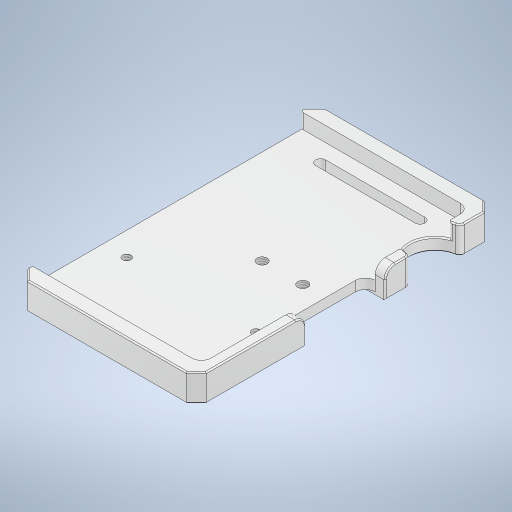
# Autodesk Inventor part: Wallet Recipe Test
Saved by Autodesk Inventor 2023.2 (Build 272271000, 271)
## iProperties
Created: 2024-03-26
Part Number: Wallet Recipe Test
Material: Aluminum 6061
Document SubType Name: Modeling
Designer: Nathan Cai
Density: 2.7 g/cm^3
Appearance: Aluminum - Flat
Author: Nathan Cai
Autodesk Inventor part; units mm, degrees
ref_plane "YZ Plane" through (0, 0, 0) normal (1, 0, 0) x (0, 1, 0)
ref_plane "XZ Plane" through (0, 0, 0) normal (0, 1, 0) x (-1, 0, 0)
ref_plane "XY Plane" through (0, 0, 0) normal (0, 0, 1) x (1, 0, 0)
sketch "Sketch1" plane through (0, 0, 0) normal (0, 1, 0) x (-1, 0, 0)
  line L0 (-28.575, 47.625) -> (28.575, 47.625)
  line L1 (28.575, 47.625) -> (28.575, -47.625)
  line L2 (28.575, -47.625) -> (-28.575, -47.625)
  line L3 (-28.575, -47.625) -> (-28.575, 47.625)
  line L4 (-28.575, 47.625) -> (28.575, -47.625) construction
  line L5 (28.575, 47.625) -> (-28.575, -47.625) construction
  point P0 (0, 0)
  dimension "d0" = 57.15
  dimension "d1" = 95.25
  constraints: 12 end point, 2 midpoint, 2 parallel, 1 horizontal, 1 perpendicular
  measures "d0" distance of L1.end L2.end
  measures "d1" distance of L0.end L1.end
extrude "Extrusion1" add sketch "Sketch1" along normal blind 8.7313
sketch "Sketch2" plane through (0, 8.7313, 0) normal (0, 1, 0) x (1, 0, 0)
  line L0 (-28.575, 47.625) -> (-28.575, -47.625) projected
  line L1 (-28.575, 0) -> (0, 0) construction
  line L2 (-28.575, -42.8625) -> (25.4, -42.8625)
  line L3 (25.4, -42.8625) -> (25.4, 42.8625)
  line L4 (25.4, 42.8625) -> (-28.575, 42.8625)
  line L5 (-28.575, 42.8625) -> (-28.575, -42.8625)
  dimension "d4" = 53.975
  dimension "d5" = 85.725
  constraints: 10 end point, 2 horizontal, 2 parallel, 1 midpoint, 1 perpendicular, 1 point on line, 1 other
  measures "d4" distance of L4.end L3.end
  measures "d5" distance of L3.end L2.end
extrude "Extrusion2" cut sketch "Sketch2" against normal blind 4.7625
fillet "Fillet1" radius 3.048 2 edges at (25.4, 6.35, 42.8625) (25.4, 6.35, -42.8625)
sketch "Sketch3" plane through (0, 0, 0) normal (0, -1, 0) x (1, 0, 0)
  line L0 (22.225, -12.7) -> (34.925, -12.7)
  line L1 (34.925, -12.7) -> (34.925, 12.7)
  line L2 (34.925, 12.7) -> (22.225, 12.7)
  line L3 (22.225, 12.7) -> (22.225, -12.7)
  line L4 (28.575, 47.625) -> (28.575, -47.625) projected
  line L5 (22.225, -12.7) -> (34.925, 12.7) construction
  line L6 (34.925, -12.7) -> (22.225, 12.7) construction
  point P0 (0, 0)
  point P1 (28.575, 0)
  dimension "d15" = 12.7
  dimension "d16" = 25.4
  constraints: 12 end point, 3 midpoint, 2 parallel, 1 horizontal, 1 perpendicular
  measures "d15" distance of L2.end L1.end
  measures "d16" distance between parallel lines of L0 L2
extrude "Extrusion3" cut sketch "Sketch3" against normal through all
sketch "Sketch4" plane through (0, 0, 0) normal (0, -1, 0) x (1, 0, 0)
  line L0 (28.575, -12.7) -> (-19.05, -12.7)
  line L1 (-19.05, -12.7) -> (-19.05, 12.7)
  line L2 (-19.05, 12.7) -> (28.575, 12.7)
  line L3 (28.575, 12.7) -> (28.575, -12.7)
  line L4 (28.575, -12.7) -> (-19.05, 12.7) construction
  line L5 (-19.05, -12.7) -> (28.575, 12.7) construction
  line L6 (0, 0) -> (22.225, 0) construction
  line L7 (22.225, 12.7) -> (22.225, -12.7) projected
  point P0 (4.7625, 0)
  point P1 (28.575, 12.7)
  point P2 (22.225, 9.525)
  point P3 (22.225, -9.525)
  dimension "d20" = 47.625
  dimension "d21" = 25.4
  constraints: 14 end point, 3 midpoint, 2 parallel, 2 point on line, 1 horizontal, 1 perpendicular
  measures "d20" distance of L1.end L2.end
  measures "d21" distance of L0.end L1.end
extrude "Extrusion4" cut sketch "Sketch4" against normal blind 0.7937
fillet "Fillet3" radius 3.175 6 edges at (22.225, 2.3813, -12.7) (26.9875, 8.7313, -12.7) (22.225, 2.3813, 12.7) (26.9875, 8.7313, 12.7) (-19.05, 0.3969, -12.7) (-19.05, 0.3969, 12.7)
sketch "Sketch5" plane through (0, 0.7937, 0) normal (0, -1, 0) x (1, 0, 0)
  line L0 (-19.05, -9.525) -> (-19.05, 9.525) projected
  line L1 (-19.05, 0) -> (22.225, 0) construction
  line L2 (22.225, 9.525) -> (22.225, -9.525) projected
  circle A0 centre (1.95, 0) radius 2
  circle A1 centre (14.95, 0) radius 2
  point P0 (0, 0)
  dimension "d25" = 4
  dimension "d26" = 21
  dimension "d29" = 13
  constraints: 2 centre point, 2 coincident, 2 end point, 2 midpoint, 1 horizontal, 1 point on line, 2 other
  measures "d25" diameter of A0
  measures "d26" distance from line of L0 A0.centre
  measures "d29" distance of A0.centre A1.centre
hole "Hole1" at (1.95, 0.7937, 0) at (14.95, 0.7937, 0) direction (0, 1, 0) diameter 3.242 end through all thread size "M4x0.7" class "6H" standard "ANSI Metric M Profile"
chamfer "Chamfer3" distance 3.175 angle 45 4 edges at (28.575, 4.3656, 47.625) (-28.575, 4.3656, 47.625) (28.575, 4.3656, -47.625) (-28.575, 4.3656, -47.625)
fillet "Fillet4" radius 0.7937 2 edges at (-28.575, 6.35, 42.8625) (-28.575, 6.35, -42.8625)
sketch "Sketch7" plane through (0, 0, 0) normal (0, -1, 0) x (1, 0, 0)
  line L0 (25.4, -47.625) -> (-25.4, -47.625) projected
  line L1 (0, -47.625) -> (0, 47.625) construction
  line L2 (-25.4, 47.625) -> (25.4, 47.625) projected
  line L3 (15.875, -36.5125) -> (-15.875, -36.5125) construction
  line L4 (15.875, -34.925) -> (-15.875, -34.925)
  line L5 (-15.875, -38.1) -> (15.875, -38.1)
  arc A0 (15.875, -38.1) -> (15.875, -34.925) centre (15.875, -36.5125) ccw
  arc A1 (-15.875, -34.925) -> (-15.875, -38.1) centre (-15.875, -36.5125) ccw
  line L6 (28.575, -12.7) -> (28.575, -44.45) projected
  circle A2 centre (28.575, -28.575) radius 7.9375
  point P0 (0, 0)
  point P1 (0, -36.5125)
  point P2 (28.575, -36.5125)
  point P3 (28.575, -20.6375)
  dimension "d50" = 3.175
  dimension "d51" = 31.75
  dimension "d52" = 9.525
  dimension "d55" = 15.875
  constraints: 10 end point, 4 midpoint, 4 point on circle, 4 tangent, 3 centre point, 1 parallel, 1 perpendicular, 1 point on line
  measures "d50" diameter of A1
  measures "d51" distance of L3.start L3.end
  measures "d52" distance between parallel lines of L0 L5
  measures "d55" diameter of A2
extrude "Extrusion6" cut sketch "Sketch7" against normal blind 25.4 contours A0 L5 A1 L4 | L6 A2 picked at (24.9577, -30.7816)
sketch "Sketch8" plane through (0, 0, 0) normal (0, -1, 0) x (1, 0, 0)
  line L0 (0, 0) -> (0, 47.625) construction
  line L1 (-25.4, 47.625) -> (25.4, 47.625) construction
  line L2 (-23.8125, 17.4625) -> (23.8125, 17.4625)
  line L3 (23.8125, 17.4625) -> (23.8125, 42.8625)
  line L4 (23.8125, 42.8625) -> (-23.8125, 42.8625)
  line L5 (-23.8125, 42.8625) -> (-23.8125, 17.4625)
  line L6 (-23.8125, 17.4625) -> (23.8125, 42.8625) construction
  line L7 (23.8125, 17.4625) -> (-23.8125, 42.8625) construction
  circle A0 centre (-20.6375, 39.6875) radius 1.7526 construction
  point P0 (0, 30.1625)
  point P1 (20.6375, 39.6875)
  point P2 (-20.6375, 20.6375)
  point P3 (20.6375, 20.6375)
  dimension "d58" = 47.625
  dimension "d59" = 25.4
  dimension "d60" = 17.4625
  dimension "d64" = 3.5052
  dimension "d65" = 3.175
  dimension "d66" = 3.175
  dimension "d79" = 41.275
  dimension "d82" = 19.05
  constraints: 14 end point, 3 midpoint, 2 horizontal, 2 parallel, 1 centre point, 1 coincident, 1 perpendicular, 1 point on line, 1 vertical, 3 other
  measures "d58" distance of L4.end L3.end
  measures "d59" distance of L3.end L2.end
  measures "d60" distance from line of L1 point (0, 30.163)
  measures "d64" diameter of A0
  measures "d65" distance from line of L4 A0.centre
  measures "d66" distance from line of L5 A0.centre
  measures "d79" distance of point (-20.638, 39.688) point (20.637, 39.688)
  measures "d82" distance of point (-20.638, 39.688) point (-20.638, 20.638)
extrude "Extrusion7" cut sketch "Sketch8" against normal blind 1.5875
fillet "Fillet7" radius 3.175 4 edges at (-23.8125, 0.7937, 17.4625) (-23.8125, 0.7937, 42.8625) (23.8125, 0.7937, 42.8625) (23.8125, 0.7937, 17.4625)
hole "Hole2" at (-20.6375, 0, 39.6875) at (20.6375, 0, 39.6875) at (-20.6375, 0, 20.6375) at (20.6375, 0, 20.6375) direction (0, 1, 0) diameter 2.6416 end through all thread size "6-32 UNC" class "2B" standard "ANSI Unified Screw Threads"
fillet "Fillet5" radius 1.5875 2 edges at (28.575, 4.3656, -36.5125) (28.575, 4.3656, -20.6375)
chamfer "Chamfer4" distance 0.3969 angle 45 32 edges at (28.575, 0, -15.9416) (28.2, 0, -20.208) (20.6375, 0, -28.575) (28.2, 0, -36.942) (28.575, 0, -41.2084) (26.9875, 0, -46.0375) (0, 0, -47.625) (-26.9875, 0, -46.0375) (-28.575, 0, 0) (-26.9875, 0, 46.0375) (0, 0, 47.625) (26.9875, 0, 46.0375) (28.575, 0, 28.575) (-26.9875, 8.7312, -46.0375) (0, 8.7313, -47.625) (26.9875, 8.7312, -46.0375) (28.575, 8.7313, -41.2084) (28.2, 8.7313, -36.942) (26.3092, 8.7313, -36.1822) (28.575, 8.7313, -17.5291) (28.2, 8.7313, -20.208) (26.3092, 8.7313, -20.9678) (28.575, 7.8013, -13.6299) (28.575, 2.7781, -12.7) (28.575, 8.7313, 30.1625) (28.575, 7.8013, 13.6299) (28.575, 2.7781, 12.7) (26.9875, 8.7312, 46.0375) (0, 8.7313, 47.625) (-26.9875, 8.7312, 46.0375) (20.6375, 3.9688, -28.575) (-28.575, 3.9688, 0)
fillet "Fillet6" radius 0.7937 4 edges at (25.4, 6.1516, -21.3002) (25.4, 3.7703, -21.3002) (25.4, 6.1516, -35.8498) (25.4, 3.7703, -35.8498)
equation "\"d66\" = d65"
equation "\"d79\" = d58 - 2 * d66"
equation "\"d82\" = d59 - 2 * d65"
body "Solid1"
